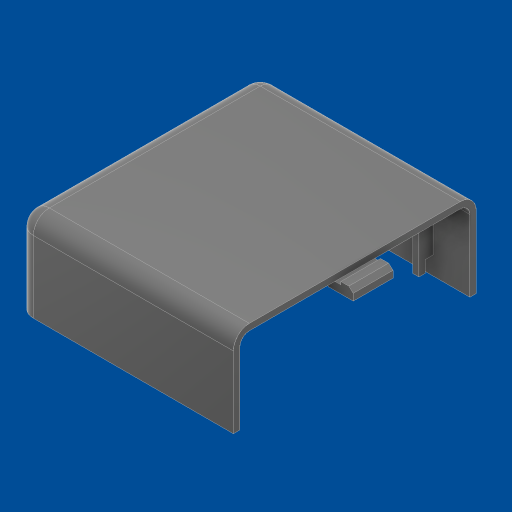
# Autodesk Inventor part: sliding_door
Saved by Autodesk Inventor 2023.2 (Build 272271000, 271)
## iProperties
Created: 2023-01-27
Part Number: sliding_door
Material: PC/ABS Plastic
Document SubType Name: Modeling
Designer: agmlego
Mass: 4.08885 g
Surface Area: 143.289 cm^2
Volume: 11.4446 cm^3
Density: 0.357273 g/cm^3
Appearance: Smooth - Black
Author: agmlego
Autodesk Inventor part; units mm, degrees
ref_plane "YZ Plane" through (0, 0, 0) normal (1, 0, 0) x (0, 1, 0)
ref_plane "XZ Plane" through (0, 0, 0) normal (0, 1, 0) x (-1, 0, 0)
ref_plane "XY Plane" through (0, 0, 0) normal (0, 0, 1) x (1, 0, 0)
sketch "Sketch1" plane through (0, 0, 0) normal (1, 0, 0) x (0, 1, 0)
  line L0 (-11, 30.5) -> (11, 30.5)
  line L1 (11, 30.5) -> (11, -30.5)
  line L2 (11, -30.5) -> (-11, -30.5)
  line L3 (-11, -30.5) -> (-11, 30.5)
  line L4 (11, 0) -> (-11, 0) construction
  point P0 (0, 0)
  point P1 (0, 0)
  dimension "d0" = 61
  dimension "d1" = 22
  constraints: 10 end point, 3 midpoint, 2 parallel, 1 coincident, 1 horizontal, 1 perpendicular
  measures "d0" distance between parallel lines of L2 L0
  measures "d1" distance between parallel lines of L3 L1
extrude "Extrusion1" add sketch "Sketch1" along normal blind 54.25
sketch "Sketch2" plane through (54.25, 0, 0) normal (1, 0, 0) x (0, 0, -1)
  line L0 (-28.9, 9.4) -> (28.9, 9.4)
  line L1 (28.9, 9.4) -> (28.9, -11)
  line L2 (28.9, -11) -> (-28.9, -11)
  line L3 (-28.9, -11) -> (-28.9, 9.4)
  line L4 (-30.5, -11) -> (30.5, -11) construction
  line L5 (-28.9, 0) -> (-30.5, 0) construction
  line L6 (0, 9.4) -> (0, 11) construction
  line L7 (30.5, 11) -> (-30.5, 11) construction
  line L8 (-30.5, 11) -> (-30.5, -11) construction
  point P0 (0, 0)
  point P1 (0, -11)
  dimension "d4" = 1.6
  constraints: 12 end point, 5 midpoint, 3 perpendicular, 2 parallel, 1 horizontal, 1 point on line
  measures "d4" distance of L6.start L6.end
extrude "Extrusion2" cut sketch "Sketch2" against normal blind 52.25
fillet "Fillet1" radius 4 5 edges at (27.125, 11, 30.5) (0, 0, 30.5) (0, 11, 0) (0, 0, -30.5) (27.125, 11, -30.5)
fillet "Fillet2" radius 2.4 5 edges at (28.125, 9.4, -28.9) (2, 9.4, 0) (2, -0.8, -28.9) (28.125, 9.4, 28.9) (2, -0.8, 28.9)
sketch "Sketch3" plane through (54.25, 9.4, -26.5) normal (0, -1, 0) x (1, 0, 0)
  line L0 (-10.7, 1.2) -> (-9.2, 1.2)
  line L1 (-9.2, 1.2) -> (-9.2, -2.4)
  line L2 (-9.2, -2.4) -> (-10.7, -2.4)
  line L3 (-10.7, -2.4) -> (-10.7, 1.2)
  line L4 (-10.7, 51.8) -> (-9.2, 51.8)
  line L5 (-9.2, 51.8) -> (-9.2, 55.4)
  line L6 (-9.2, 55.4) -> (-10.7, 55.4)
  line L7 (-10.7, 55.4) -> (-10.7, 51.8)
  line L8 (0, -2.4) -> (-49.85, -2.4) construction
  line L9 (-49.85, 55.4) -> (0, 55.4) construction
  line L10 (0, 53) -> (0, 0) construction
  point P0 (-54.25, 26.5)
  dimension "d29" = 1.5
  dimension "d30" = 9.2
  dimension "d31" = 50.6
  constraints: 16 end point, 4 parallel, 3 collinear, 2 horizontal, 2 perpendicular, 2 point on line
  measures "d29" distance of L4.start L4.end
  measures "d30" distance between parallel lines of L10 L5
  measures "d31" distance between parallel lines of L0 L4
sketch "Sketch4" plane through (0, 0, 0) normal (0, 0, 1) x (1, 0, 0)
  line L0 (52.65, 7.4) -> (58.85, 7.4)
  line L1 (58.85, 7.4) -> (58.85, 10.0442)
  line L2 (55.73, 9.4) -> (52.65, 9.4)
  line L3 (52.65, 9.4) -> (52.65, 7.4)
  line L4 (55.73, 9.4) -> (55.73, 10.1)
  line L5 (55.73, 10.1) -> (58.85, 10.1)
  line L6 (58.85, 10.1) -> (58.85, 10.0442)
  point P0 (0, 0)
  point P1 (54.25, 9.4)
  dimension "d9" = 2.7
  dimension "d10" = 2
  dimension "d11" = 6.2
  dimension "d12" = 3.12
  dimension "d13" = 4.6
  constraints: 14 end point, 4 parallel, 1 horizontal, 1 perpendicular, 1 point on line
  measures "d9" distance between parallel lines of L5 L0
  measures "d10" distance of L2.end L0.start
  measures "d11" distance of L0.start L0.end
  measures "d12" distance of L4.end L5.end
  measures "d13" distance from line of point (54.25, 9.4) L1
extrude "Extrusion3" add sketch "Sketch4" along normal mid plane 10
sketch "Sketch5" plane through (4.4, 9.4, 26.5) normal (0, -1, 0) x (1, 0, 0)
  line L0 (48.25, -31.5) -> (48.25, -21.5) construction
  line L1 (48.25, -21.5) -> (45.83, -21.5)
  line L2 (45.83, -21.5) -> (45.83, -22.64)
  line L3 (45.83, -22.64) -> (48.25, -22.64)
  line L4 (48.25, -22.64) -> (48.25, -21.5)
  line L5 (48.25, -31.5) -> (45.83, -31.5)
  line L6 (45.83, -31.5) -> (45.83, -30.36)
  line L7 (45.83, -30.36) -> (48.25, -30.36)
  line L8 (48.25, -30.36) -> (48.25, -31.5)
  line L9 (54.45, -31.5) -> (54.45, -21.5) construction
  point P0 (-4.4, -26.5)
  dimension "d16" = 1.14
  dimension "d17" = 8.62
  constraints: 16 end point, 4 parallel, 2 horizontal, 2 perpendicular, 1 collinear, 1 point on line
  measures "d16" distance of L1.end L2.end
  measures "d17" distance between parallel lines of L9 L2
extrude "Extrusion4" add sketch "Sketch5" along normal up to surface (2 mm away)
chamfer "Chamfer1" distance 2 distance2 2.42 1 edges at (50.23, 7.4, -4.43) measured on face at (50.23, 8.7333, -4.24)
chamfer "Chamfer2" distance 2 distance2 2.42 1 edges at (50.23, 7.4, 4.43) measured on face at (50.23, 8.0667, 4.24)
chamfer "Chamfer3" distance 1 distance2 1.12 1 edges at (58.85, 10.1, 0) measured on face at (58.85, 8.3, -1.6667)
extrude "Extrusion5" add sketch "Sketch3" along normal blind 18.8
sketch "Sketch6" plane through (45.05, 9.4, -25.3) normal (1, 0, 0) x (0, 0, -1)
  line L0 (3.6, -18.8) -> (0, -18.8) construction
  line L1 (3.6, -18.8) -> (1.6, -18.8)
  line L2 (1.6, -18.8) -> (1.6, -15.8)
  line L3 (1.6, -15.8) -> (3.6, -15.8)
  line L4 (3.6, -15.8) -> (3.6, -18.8)
  line L5 (-54.2, -18.8) -> (-50.6, -18.8) construction
  line L6 (-54.2, -18.8) -> (-52.2, -18.8)
  line L7 (-52.2, -18.8) -> (-52.2, -15.8)
  line L8 (-52.2, -15.8) -> (-54.2, -15.8)
  line L9 (-54.2, -15.8) -> (-54.2, -18.8)
  line L10 (0, 0) -> (0, -18.8) construction
  point P0 (-25.3, -9.4)
  dimension "d35" = 1.6
  dimension "d36" = 3
  constraints: 16 end point, 4 parallel, 2 equal length, 2 horizontal, 2 perpendicular
  measures "d35" distance between parallel lines of L10 L2
  measures "d36" distance of L1.end L2.end
extrude "Extrusion6" cut sketch "Sketch6" against normal up to surface (1.5 mm away)
sketch "Sketch7" plane through (4.4, 9.4, -26.5) normal (0, -1, 0) x (1, 0, 0)
  line L0 (-2.4, 53) -> (-2.4, 0) construction
  line L1 (-2.4, 13.4) -> (25.5, 13.4)
  line L2 (25.5, 13.4) -> (25.5, 14.6)
  line L3 (25.5, 14.6) -> (-2.4, 14.6)
  line L4 (-2.4, 14.6) -> (-2.4, 13.4)
  line L5 (-2.4, 39.6) -> (25.5, 39.6)
  line L6 (25.5, 39.6) -> (25.5, 38.4)
  line L7 (25.5, 38.4) -> (-2.4, 38.4)
  line L8 (-2.4, 38.4) -> (-2.4, 39.6)
  line L9 (25.5, 14.6) -> (25.5, 38.4) construction
  line L10 (25.5, 26.5) -> (-4.4, 26.5) construction
  dimension "d39" = 1.2
  dimension "d40" = 23.8
  dimension "d41" = 27.9
  constraints: 20 end point, 4 parallel, 3 perpendicular, 2 collinear, 2 horizontal, 2 point on line, 1 midpoint, 1 vertical
  measures "d39" distance of L1.end L2.end
  measures "d40" distance between parallel lines of L7 L3
  measures "d41" distance of L1.start L1.end
extrude "Extrusion7" add sketch "Sketch7" along normal blind 3.75
sketch "Sketch8" plane through (4.4, 5.65, -26.5) normal (0, -1, 0) x (1, 0, 0)
  line L0 (-2.4, 0) -> (-2.4, 53) construction
  line L1 (0, 14.6) -> (25.5, 14.6) construction
  line L2 (-2.4, 13.4) -> (7.35, 13.4)
  line L3 (7.35, 13.4) -> (7.35, 14.6)
  line L4 (7.35, 14.6) -> (-2.4, 14.6)
  line L5 (-2.4, 14.6) -> (-2.4, 13.4)
  line L6 (-2.4, 38.4) -> (-2.4, 39.6) construction
  line L7 (-2.4, 38.4) -> (25.5, 38.4) construction
  line L8 (-2.4, 39.6) -> (7.35, 39.6)
  line L9 (7.35, 39.6) -> (7.35, 38.4)
  line L10 (7.35, 38.4) -> (-2.4, 38.4)
  line L11 (-2.4, 38.4) -> (-2.4, 39.6)
  line L12 (-2.4, 13.4) -> (25.5, 13.4) construction
  point P0 (-4.4, 26.5)
  dimension "d44" = 9.75
  constraints: 16 end point, 4 parallel, 3 point on line, 2 collinear, 2 horizontal, 2 perpendicular
  measures "d44" distance between parallel lines of L0 L3
extrude "Extrusion8" add sketch "Sketch8" along normal blind 4.5
fillet "Fillet3" radius 2 2 edges at (29.9, 5.65, 12.5) (29.9, 5.65, -12.5)
sketch "Sketch9" plane through (2, 0, 0) normal (1, 0, 0) x (0, 0, -1)
  line L0 (-26.5, -11) -> (26.5, -11) construction
  line L1 (22.5, -11) -> (17.5, -11)
  line L2 (17.5, -11) -> (17.5, -9.77)
  line L3 (17.5, -9.77) -> (22.5, -9.77)
  line L4 (22.5, -9.77) -> (22.5, -11)
  line L5 (-22.5, -11) -> (-17.5, -11)
  line L6 (-17.5, -11) -> (-17.5, -9.77)
  line L7 (-17.5, -9.77) -> (-22.5, -9.77)
  line L8 (-22.5, -9.77) -> (-22.5, -11)
  line L9 (17.5, -9.77) -> (-17.5, -9.77) construction
  line L10 (0, -9.77) -> (0, -11) construction
  point P0 (0, 0)
  dimension "d48" = 5
  dimension "d49" = 35
  dimension "d50" = 1.23
  constraints: 20 end point, 4 parallel, 3 horizontal, 3 perpendicular, 3 point on line, 2 midpoint, 1 collinear
  measures "d48" distance of L2.end L3.end
  measures "d49" distance of L2.end L6.end
  measures "d50" distance of L3.end L1.start
extrude "Extrusion9" add sketch "Sketch9" along normal blind 3
body "Solid1"
